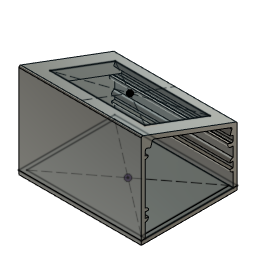
OctoCase (Autodesk Fusion 360 design; units mm, degrees)
Autodesk Fusion 360 part; units mm, degrees
sketch "Sketch1" plane through (0, 0, 0) normal (0, 0, 1) x (1, 0, 0) in component "Case"
  line L0 (17.2, -13.2) -> (-17.2, -13.2)
  line L1 (-17.2, -13.2) -> (-17.2, 13.2)
  line L2 (-17.2, 13.2) -> (17.2, 13.2)
  line L3 (17.2, 13.2) -> (17.2, -13.2)
  line L4 (17.2, -13.2) -> (-17.2, 13.2) construction
  line L5 (-17.2, -13.2) -> (17.2, 13.2) construction
  line L6 (-18.4, -14.4) -> (-18.4, 14.4)
  line L7 (-18.4, 14.4) -> (18.4, 14.4)
  line L8 (18.4, 14.4) -> (18.4, -14.4)
  line L9 (18.4, -14.4) -> (-18.4, -14.4)
  line L10 (17.2, 13.2) -> (18.4, 13.2)
  line L11 (17.2, -13.2) -> (18.4, -13.2)
  dimension "d8" = 34.4
  dimension "d9" = 26.4
  constraint horizontal L0
  constraint perpendicular L0 L1
  constraint parallel L0 L2
  constraint parallel L1 L3
  constraint coincident L4 origin
  constraint coincident L5 origin
  constraint coincident L8 L10.end
  constraint perpendicular L8 L10
  constraint coincident L8 L11.end
  constraint perpendicular L8 L11
  measures "d8" distance of L1.end L2.end
  measures "d9" distance of L0 L2
extrude "Extrude1" add sketch "Sketch1" along normal blind 11.9 contours L0 L1 L2 L6 L7 L8 L9 L10 L11 in component "Case"
extrude "Extrude2" add sketch "Sketch1" against normal blind 1.2 in component "Case"
sketch "Sketch2" plane through (-17.2, 0, 0) normal (1, 0, 0) x (0, 1, 0) in component "Case"
  line L0 (-13.2, 0) -> (13.2, 0)
  line L1 (13.2, 0) -> (13.2, 11.9)
  line L2 (13.2, 11.9) -> (-13.2, 11.9)
  line L3 (-13.2, 11.9) -> (-13.2, 0)
  line L4 (14.4, 0) -> (-14.4, 0)
  line L5 (0, 2.5) -> (0, 20)
  line L6 (13.2, 5.2) -> (-13.2, 5.2)
  line L7 (-13.2, 5.2) -> (-13.2, 6.9) construction
  line L8 (-13.2, 6.9) -> (13.2, 6.9)
  line L9 (13.2, 6.9) -> (13.2, 5.2) construction
  line L10 (13.2, 5.2) -> (-13.2, 6.9) construction
  line L11 (-13.2, 5.2) -> (13.2, 6.9) construction
  circle A0 centre (-13.2, 5.2) radius 1
  circle A1 centre (-13.2, 6.9) radius 1
  circle A2 centre (13.2, 6.9) radius 1
  circle A3 centre (13.2, 5.2) radius 1
  line L12 (13.2, 13.5869) -> (-12.572, 23.1814)
  line L13 (-12.572, 23.1814) -> (-13.2, 21.4945) construction
  line L14 (-13.2, 21.4945) -> (12.572, 11.9) construction
  line L15 (12.572, 11.9) -> (13.2, 13.5869) construction
  line L16 (-13.2, 11.9) -> (-13.2, 27.5) construction
  line L17 (13.2, 11.9) -> (13.2, 20.1316) construction
  line L18 (12.572, 11.9) -> (12.8, 11.9)
  line L19 (14.4, 0) -> (14.4, 20.1451) construction
  line L20 (13.2, 13.5869) -> (14.4, 13.5869)
  line L21 (14.4, 16.2768) -> (14.4, 11.65)
  line L22 (14.4, 11.65) -> (13.2, 11.65)
  line L23 (13.2, 12.3) -> (13.2, 13.5869)
  circle A4 centre (12.572, 11.9) radius 1
  line L24 (13.2, 10.9) -> (12.572, 10.9)
  line L25 (-14.4, 0) -> (-14.4, 28) construction
  circle A5 centre (-12.572, 23.1814) radius 1
  circle A6 centre (13.2, 13.5869) radius 1
  line L26 (-10.5622, 24.5673) -> (12.5858, 15.9497)
  line L27 (14.4, 13.5869) -> (14.4, 15.2743)
  circle A7 centre (-13.2, 21.4945) radius 1
  line L28 (-14.4, 26.7007) -> (-14.4, 0)
  line L29 (-13.2, 11.9) -> (-13.2, 22.8394)
  line L30 (11.6348, 12.2489) -> (12.572, 11.9)
  line L31 (13.2, 13.5869) -> (12.2628, 13.9358)
  line L32 (-13.2, 21.4945) -> (-12.2628, 21.1456)
  line L33 (-12.572, 23.1814) -> (-11.6348, 22.8325)
  line L34 (-12.572, 23.1814) -> (-12.6604, 23.2143)
  arc A8 (-12.6604, 23.2143) -> (-13.2, 22.8394) centre (-12.8, 22.8394) ccw
  arc A9 (12.8, 11.9) -> (13.2, 12.3) centre (12.8, 12.3) ccw
  line L35 (-13.8604, 27.0756) -> (14.1396, 16.6517)
  line L36 (-11.6348, 22.8325) -> (-11.0766, 24.332)
  arc A10 (-10.5622, 24.5673) -> (-11.0766, 24.332) centre (-10.7017, 24.1924) ccw
  line L37 (12.2628, 13.9358) -> (12.8211, 15.4352)
  arc A11 (12.8211, 15.4352) -> (12.5858, 15.9497) centre (12.4462, 15.5748) ccw
  arc A12 (14.4, 16.2768) -> (14.1396, 16.6517) centre (14, 16.2768) ccw
  arc A13 (-13.8604, 27.0756) -> (-14.4, 26.7007) centre (-14, 26.7007) ccw
  point P0 (0, 6.05)
  point P1 (-14.4, 27.2765)
  dimension "d32" = 1.7
  dimension "d33" = 5.2
  dimension "d35" = 2
  dimension "d36" = 2
  dimension "d37" = 2
  dimension "d38" = 2
  dimension "d39" = 27.5
  dimension "d40" = 1.8
  dimension "d41" = 2
  dimension "d42" = 2
  dimension "d43" = 2
  dimension "d44" = 2
  dimension "d47" = 0.4
  dimension "d48" = 0.4
  dimension "d54" = 1.2
  dimension "d55" = 0.4
  dimension "d56" = 0.4
  dimension "d57" = 0.4
  dimension "d58" = 0.4
  dimension "d63" = 2
  constraint horizontal L6
  constraint perpendicular L6 L7
  constraint parallel L6 L8
  constraint parallel L7 L9
  constraint coincident L1 L6.start
  constraint coincident L10 P0
  constraint coincident L11 P0
  constraint coincident L5 P0
  constraint coincident L6.end L7.start
  constraint coincident L7.end L8.start
  constraint coincident L8.end L9.start
  constraint coincident L6.start L9.end
  constraint perpendicular L12 L13
  constraint parallel L12 L14
  constraint parallel L13 L15
  constraint coincident L2.end L3.start
  constraint perpendicular L2 L16
  constraint coincident L13.end L16
  constraint coincident L1.end L2.start
  constraint perpendicular L2 L17
  constraint coincident L12.start L17
  constraint perpendicular L17 L18
  constraint coincident L4.start L19.start
  constraint perpendicular L4 L19
  constraint horizontal L20
  constraint vertical L21
  constraint horizontal L22
  constraint vertical L23
  constraint coincident L19 L21.end
  constraint coincident L14.end L15.start
  constraint coincident L1 L24.start
  constraint coincident A4 L24.end
  constraint tangent A4 L24
  constraint perpendicular L1 L24
  constraint coincident L4.end L25.start
  constraint perpendicular L4 L25
  constraint coincident L12.end L13.start
  constraint coincident L12.start L15.end
  constraint coincident L19 L27.end
  constraint parallel L12 L26
  constraint coincident L13.end L14.start
  constraint coincident A4 L30.start
  constraint coincident L14 L30.start
  constraint coincident A6 L31.end
  constraint coincident L12 L31.end
  constraint coincident A7 L32.end
  constraint coincident L14 L32.end
  constraint coincident A5 L33.end
  constraint coincident L12 L33.end
  constraint collinear L12 L34
  constraint coincident L27.end L26
  constraint coincident L20.end L21
  constraint tangent L29 A8
  constraint tangent L34 A8
  constraint coincident L22.end L23
  constraint tangent L23 A9
  constraint tangent L18 A9
  constraint collinear L25 L28
  constraint coincident L25 P1
  constraint parallel L26 L35
  constraint collinear L2 L18
  constraint collinear L16 L29
  constraint tangent A5 L36
  constraint tangent L36 A10
  constraint tangent L26 A10
  constraint tangent A6 L37
  constraint tangent L37 A11
  constraint tangent L26 A11
  constraint tangent L35 A12
  constraint tangent L21 A12
  constraint coincident P1 L35
  constraint tangent L28 A13
  constraint tangent L35 A13
  measures "d32" distance of L6 L8
  measures "d33" distance of L4 L6
  measures "d35" diameter of A0
  measures "d36" diameter of A1
  measures "d37" diameter of A2
  measures "d38" diameter of A3
  measures "d39" distance of L12.start L12.end
  measures "d40" distance of L12.end L13.end
  measures "d41" diameter of A4
  measures "d42" diameter of A5
  measures "d43" diameter of A6
  measures "d44" diameter of A7
  measures "d47" radius of A8
  measures "d48" radius of A9
  measures "d54" distance of L26 P1
  measures "d55" radius of A10
  measures "d56" radius of A11
  measures "d57" radius of A12
  measures "d58" radius of A13
  measures "d63" distance of L12 L26
extrude "Extrude4" add sketch "Sketch2" along normal up to surface (35.6 mm away) contours L3 L4 A0 A1 L20 L21 A5 A6 L26 L27 A7 L28 L29 L35 L36 A10 L37 A11 A12 A13 | L3 L6 A0 | L1 L6 A3 | L3 L8 A1 | L1 L8 A2 | A7 L29 L32 | A5 A7 L29 | L2 A4 L30 | L1 L2 L18 A4 | A5 A7 L29 | L12 A5 A7 L29 L33 L34 A8 | L1 A4 L24 | L12 L20 A6 L31 | L20 L21 L22 A4 A6 | L1 L22 A4 | L1 L2 L22 L23 A4 A6 A9 | L20 L23 A4 A6 | L23 A4 A6 picked at (-13.3251, 22.1063) picked at (-13.2109, 22.4428) picked at (-13.2727, 22.6449) picked at (13.2109, 12.6386) in component "Case"
extrude "Extrude5" add sketch "Sketch2" against normal blind 1.2 contours L3 L4 A0 A1 L20 L21 A5 A6 L26 L27 A7 L28 L29 L35 L36 A10 L37 A11 A12 A13 | L2 L5 L12 A5 A7 L29 | L2 L5 L12 A4 A6 | A7 L29 L32 | A5 A7 L29 | L2 A4 L30 | L1 L2 L18 A4 | L12 L26 L36 A10 L37 A11 | A5 A7 L29 | L12 A5 A7 L29 L33 L34 A8 | A5 A7 L29 L32 | L2 L18 L23 A4 A6 L30 A9 | L12 L20 A6 L31 | L12 L23 A4 A6 L31 | L12 A5 A7 L29 L33 L34 A8 | A5 A7 L29 | L20 L21 L22 A4 A6 | L1 L22 A4 | L1 L2 L22 L23 A4 A6 A9 | L23 A4 A6 | L20 L23 A4 A6 | L23 A4 A6 in component "Case"
sketch "Sketch5" plane through (0, 7.1657, 19.2479) normal (0, 0.34889, 0.937164) x (-1, 0, 0) in component "Case"
  line L0 (-18.4, 22.4359) -> (-18.4, -7.4415)
  line L1 (-18.4, -7.4415) -> (18.4, -7.4415)
  line L2 (18.4, -7.4415) -> (18.4, 22.4359)
  line L3 (18.4, 22.4359) -> (-18.4, 22.4359)
  line L4 (14.25, -3.4415) -> (-14.25, -3.4415)
  line L5 (-14.25, -3.4415) -> (-14.25, 17.4359)
  line L6 (-14.25, 17.4359) -> (14.25, 17.4359)
  line L7 (14.25, 17.4359) -> (14.25, -3.4415)
  line L8 (14.25, -3.4415) -> (-14.25, 17.4359) construction
  line L9 (-14.25, -3.4415) -> (14.25, 17.4359) construction
  line L10 (0, 22.4359) -> (0, -7.4415) construction
  point P0 (0, 6.9972)
  dimension "d59" = 28.5
  dimension "d64" = 4
  dimension "d65" = 5
  constraint horizontal L4
  constraint perpendicular L4 L5
  constraint parallel L4 L6
  constraint parallel L5 L7
  constraint coincident L8 P0
  constraint coincident L9 P0
  constraint midpoint L3 L10.start
  constraint midpoint L1 L10.end
  constraint coincident P0 L10
  measures "d59" distance of L5.end L6.end
  measures "d64" distance of L1 L4
  measures "d65" distance of L3 L6
extrude "Extrude6" cut sketch "Sketch5" against normal up to surface (1.2 mm away) contours L4 L5 L6 L7 in component "Case"
extrude "Extrude7" add sketch "Sketch2" along normal up to surface (2.95 mm away) contours L12 L26 L36 A10 L37 A11 in component "Case"
component "Case" placed x (1, 0, 0) y (0, 1, 0) z (0, 0, 1) at (0, 0, 0)
equation "pcb_width = 26 mm"
equation "pcb_length = 34 mm"
equation "pcb_height = 1.5 mm"
equation "pcb_clearance_top = 5 mm"
equation "pcb_clearance_bottom = 5 mm"
equation "case_gap = 0.2 mm"
equation "case_wall = 1.2 mm"
equation "d8 = pcb_length + 2 * case_gap"
equation "d9 = pcb_width + 2 * case_gap"
equation "d10 = -case_wall"
equation "d11 = 2 * case_gap + pcb_clearance_bottom + pcb_height + pcb_clearance_top"
equation "d13 = -case_wall"
equation "d32 = pcb_height + case_gap"
equation "d33 = pcb_clearance_bottom + case_gap"
equation "d36 = d35"
equation "d37 = d35"
equation "d38 = d35"
equation "d40 = 1.6 mm + case_gap"
equation "d41 = d35"
equation "d42 = d35"
equation "d43 = d35"
equation "d44 = d35"
equation "d49 = -case_wall"
equation "d54 = case_wall"
